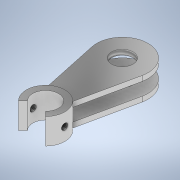
# Autodesk Inventor part: KEP_BUT
Saved by Autodesk Inventor 2022 (Build 260153000, 153)
## iProperties
Created: 2022-11-18
Part Number: KEP_BUT
Material: Nickel-Copper Alloy 400
Document SubType Name: Modeling
Designer: nguye
Density: 8.83 g/cm^3
Appearance: Chrome - Polished
Author: nguye
Autodesk Inventor part; units mm, degrees
sketch "Sketch1" plane through (0, 0, 0) normal (0, 1, 0) x (-1, 0, 0)
  circle A0 centre (0, 0) radius 5
  circle A1 centre (0, 0) radius 7.5
  dimension "d0" = 10
  dimension "d1" = 15
  constraints: 2 centre point, 2 coincident
  measures "d0" diameter of A0
  measures "d1" diameter of A1
extrude "Extrusion1" add sketch "Sketch1" along normal blind 10
ref_plane "Work Plane1" through (0, 7.5, 0) normal (0, 1, 0) x (1, 0, 0)
sketch "Sketch2" plane through (0, 7.5, 0) normal (0, 1, 0) x (1, 0, 0)
  line L0 (-5, 5.5902) -> (-5, 15)
  line L1 (-5, 15) -> (5, 15)
  line L2 (5, 15) -> (5, 5.5902)
  circle A0 centre (0, 0) radius 7.5 projected
  circle A1 centre (0, 0) radius 7.5 projected
  dimension "d5" = 10
  dimension "d6" = 5
  dimension "d7" = 15
  constraints: 6 end point, 2 perpendicular, 1 point on circle, 1 vertical, 2 other
  measures "d5" distance of L0.end L1.end
  measures "d6" distance from line of point (0, 0) L0
  measures "d7" distance from line of point (0, 0) L1
extrude "Extrusion2" add sketch "Sketch2" along normal blind 2 contours L0 L1 L2 A0
ref_plane "Work Plane2" through (0, 5, 0) normal (0, -1, 0) x (1, 0, 0)
sketch "Sketch4" plane through (0, 7.5, 0) normal (0, -1, 0) x (1, 0, 0)
  circle A0 centre (0, -30) radius 10
  line L0 (5, -5.5902) -> (5, -15) projected
  line L1 (-5, -15) -> (-5, -5.5902) projected
  line L2 (-5, -5.5902) -> (-9.7784, -27.9062)
  line L3 (5, -5.5902) -> (9.7784, -27.9062)
  line L4 (5, -15) -> (-5, -15) projected
  point P0 (0, 0)
  dimension "d11" = 20
  dimension "d26" = 30
  constraints: 4 end point, 2 point on circle, 2 tangent, 1 centre point, 1 vertical alignment
  measures "d11" diameter of A0
  measures "d26" distance of point (0, 0) A0.centre
sketch "Sketch5" plane through (0, 10, 0) normal (0, 1, 0) x (1, 0, 0)
  line L0 (0, 0) -> (-8, -8)
  line L1 (-8, -8) -> (8, -8)
  line L2 (8, -8) -> (0, 0)
  line L3 (-13.7421, 0) -> (14.2579, 0) projected
  dimension "d12" = 8
  dimension "d13" = 45
  dimension "d14" = 45
  constraints: 6 end point, 1 perpendicular
  measures "d12" horizontal distance of L1.end L0.start
  measures "d13" angle of L3 L2
  measures "d14" angle of L3 L0
extrude "Extrusion3" cut sketch "Sketch5" against normal blind 10
ref_plane "Work Plane3" through (7.5, 0, 0) normal (1, 0, 0) x (0, 1, 0)
sketch "Sketch6" plane through (7.5, 0, 0) normal (1, 0, 0) x (0, 1, 0)
  point P0 (0, 0)
  point P1 (5, 0)
  dimension "d18" = 5
  constraints: 1 horizontal alignment
  measures "d18" distance of point (0, 0) point (5, 0)
hole "Hole1" at (7.5, 5, 0) direction (-1, 0, 0) diameter 2.459 end through all thread size "M3x0.5" class "6H" standard "ISO Metric profile"
extrude "Extrusion4" add sketch "Sketch4" against normal blind 2
ref_plane "Work Plane5" through (0, 5, 0) normal (0, -1, 0) x (1, 0, 0)
mirror "Mirror2" about plane through (0, 5, 0) normal (0, -1, 0) of "Extrusion2", "Extrusion4"
sketch "Sketch7" plane through (0, 9.5, 0) normal (0, 1, 0) x (1, 0, 0)
  arc A0 (9.7784, 27.9062) -> (-9.7784, 27.9062) centre (0, 30) ccw projected
  point P0 (0, 0)
  constraints: 1 coincident
hole "Hole2" at (0, 9.5, -30) direction (0, -1, 0) diameter 8.376 end through all thread size "M10x1.5" class "6H" standard "ISO Metric profile"
body "Solid1"
